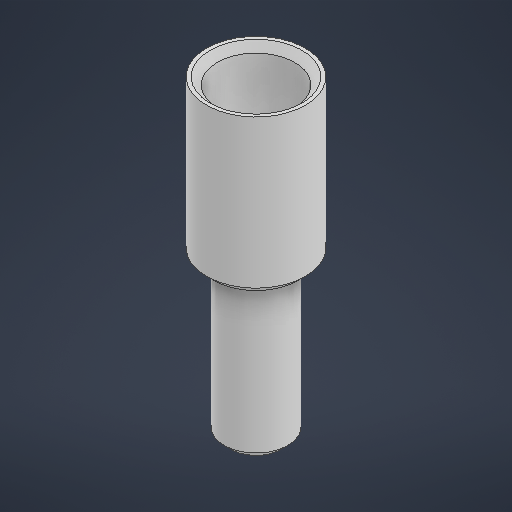
# Autodesk Inventor part: connector
Saved by Autodesk Inventor 2025.1 (Build 291241000, 241)
## iProperties
Created: 2025-11-25
Part Number: connector
Material: Типовые
Document SubType Name: Modeling
Designer: bogda
Density: 1 g/cm^3
Appearance: По умолчанию
Author: bogda
Autodesk Inventor part; units mm, degrees
ref_plane "YZ Plane" through (0, 0, 0) normal (1, 0, 0) x (0, 1, 0)
ref_plane "XZ Plane" through (0, 0, 0) normal (0, 1, 0) x (-1, 0, 0)
ref_plane "XY Plane" through (0, 0, 0) normal (0, 0, 1) x (1, 0, 0)
sketch "Эскиз1" plane through (0, 0, 0) normal (0, 1, 0) x (-1, 0, 0)
  circle A0 centre (0, 0) radius 2.25
  circle A1 centre (0, 0) radius 2.75
  circle A2 centre (0, 0) radius 3.5
  dimension "d0" = 4.5
  dimension "d1" = 5.5
  dimension "d2" = 7
  constraints: 3 centre point, 3 coincident
  measures "d0" diameter of A0
  measures "d1" diameter of A1
  measures "d2" diameter of A2
extrude "Выдавливание1" add sketch "Эскиз1" against normal blind 4 contours A0 | A1 | A2
extrude "Выдавливание2" add sketch "Эскиз1" against normal blind 15 contours A0
extrude "Выдавливание3" add sketch "Эскиз1" along normal blind 7 contours A2
chamfer "Фаска1" distance 0.5 angle 45 3 edges at (3.5, -4, 0) (2.25, -15, 0) (2.75, 7, 0)
